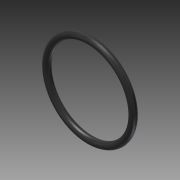
# Autodesk Inventor part: OringBig
Saved by Autodesk Inventor 2014 SP2 (Build 180246200, 246)
## iProperties
Created: 2015-09-18
Part Number: OringBig
Material: Rubber
Document SubType Name: Modeling
Designer: Lukasz Szmit
Density: 0.93 g/cm^3
Appearance: Rubber - Black - Version 1.1
Author: Lukasz Szmit
Autodesk Inventor part; units mm, degrees
ref_plane "YZ Plane" through (0, 0, 0) normal (1, 0, 0) x (0, 1, 0)
ref_plane "XZ Plane" through (0, 0, 0) normal (0, 1, 0) x (-1, 0, 0)
ref_plane "XY Plane" through (0, 0, 0) normal (0, 0, 1) x (1, 0, 0)
sketch "Sketch1" plane through (0, 0, 0) normal (0, 0, 1) x (1, 0, 0)
  circle A0 centre (-13, 0.3699) radius 1
  line L0 (0, -1.0301) -> (0, 1.7699) projected
  point P0 (0, 0)
  dimension "d0" = 2
  dimension "d1" = 13
  constraints: 1 centre point
  measures "d0" diameter of A0
  measures "d1" horizontal distance of point (0, 0) A0.centre
revolve "Revolution1" add sketch "Sketch1" angle 360 about axis through (0, -10, 0) along (0, 1, 0)
body "Solid1"
